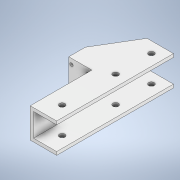
# Autodesk Inventor part: Soporte Linear Rail X
Saved by Autodesk Inventor 2021 (Build 250183000, 183)
## iProperties
Created: 2023-01-21
Part Number: Soporte Linear Rail X
Material: Plástico ABS
Document SubType Name: Modeling
Designer: Diego.labarca
Density: 1.06 g/cm^3
Appearance: Suave - Blanco
Author: Diego.labarca
Autodesk Inventor part; units mm, degrees
ref_plane "YZ Plane" through (0, 0, 0) normal (1, 0, 0) x (0, 1, 0)
ref_plane "XZ Plane" through (0, 0, 0) normal (0, 1, 0) x (-1, 0, 0)
ref_plane "XY Plane" through (0, 0, 0) normal (0, 0, 1) x (1, 0, 0)
sketch "Boceto1" plane through (0, 0, 0) normal (0, 0, 1) x (1, 0, 0)
  line L0 (-10, 11) -> (10, 11)
  line L1 (10, 11) -> (10, -11)
  line L2 (10, -11) -> (-10, -11)
  line L3 (-10, -11) -> (-10, 11)
  line L4 (1.6972, 0) -> (0, 0)
  line L5 (0, 0) -> (0, 1.3941)
  dimension "d11" = 22
  dimension "d12" = 20
  constraints: 12 end point, 2 horizontal, 2 parallel, 2 perpendicular, 2 other
  measures "d11" distance of L0.end L1.end
  measures "d12" distance of L0.start L0.end
extrude "Extrusión1" add sketch "Boceto1" along normal blind 15
sketch "Boceto5" plane through (0, 0, 15) normal (0, 0, 1) x (1, 0, 0)
  line L0 (-10, -11) -> (10, -11) projected
  line L1 (-10, -11) -> (35, -11)
  line L2 (35, -11) -> (35, -14)
  line L3 (35, -14) -> (-10, -14)
  line L4 (-10, -14) -> (-10, -11)
  line L5 (10, -11) -> (10, 11) projected
  line L6 (-10, 11) -> (-10, -11) projected
  line L7 (-10, 10) -> (35, 10)
  line L8 (35, 10) -> (35, 13)
  line L9 (35, 13) -> (-10, 13)
  line L10 (-10, 13) -> (-10, 10)
  line L11 (10, 11) -> (-10, 11) projected
  point P0 (0, 0)
  point P1 (10, 10)
  dimension "d25" = 3
  dimension "d26" = 25
  dimension "d28" = 3
  dimension "d29" = 1
  constraints: 16 end point, 4 parallel, 2 horizontal, 2 perpendicular, 1 collinear, 1 point on line
  measures "d25" distance of L1.end L2.end
  measures "d26" distance between parallel lines of L5 L2
  measures "d28" distance of L8.end L7.end
  measures "d29" distance from line of L7.start L11
extrude "Extrusión5" add sketch "Boceto5" against normal up to surface (15 mm away) contours L0 L1 L2 L3 L4 | L5 L11 L10 L9 L8 L7
sketch "Boceto7" plane through (0, 0, 0) normal (0, 0, -1) x (-1, 0, 0)
  line L0 (10, 13) -> (-35, 13) projected
  line L1 (-35, 10) -> (-10, 10) projected
  line L2 (-35, 13) -> (-15, 13)
  line L3 (-15, 13) -> (-15, 10)
  line L4 (-15, 10) -> (-35, 10)
  line L5 (-35, 10) -> (-35, 13)
  line L6 (-10, -11) -> (-35, -11) projected
  line L7 (-35, -14) -> (10, -14) projected
  line L8 (-35, -11) -> (-15, -11)
  line L9 (-15, -11) -> (-15, -14)
  line L10 (-15, -14) -> (-35, -14)
  line L11 (-35, -14) -> (-35, -11)
  point P0 (0, 0)
  dimension "d32" = 20
  constraints: 16 end point, 4 parallel, 3 point on line, 2 horizontal, 2 perpendicular
  measures "d32" distance of L3.end L4.end
extrude "Extrusión6" add sketch "Boceto7" along normal blind 35 and the other way blind 71
ref_plane "Plano de trabajo1" through (0, 0, 7.5) normal (0, 0, -1) x (-1, 0, 0)
sketch "Boceto10" plane through (0, 0, -35) normal (0, 0, -1) x (-1, 0, 0)
  line L0 (10, 13) -> (-15, 13) projected
  line L1 (-10, 10) -> (-15, 10) projected
  line L2 (-15, 13) -> (-14, 13)
  line L3 (-14, 13) -> (-14, 10)
  line L4 (-14, 10) -> (-15, 10)
  line L5 (-15, 10) -> (-15, 13)
  line L6 (-15, -14) -> (-15, -11) projected
  line L7 (10, -14) -> (-15, -14) projected
  line L8 (-15, -11) -> (-14, -11)
  line L9 (-14, -11) -> (-14, -14)
  line L10 (-14, -14) -> (-15, -14)
  line L11 (-15, -14) -> (-15, -11)
  line L12 (-14, -14) -> (-11, -14)
  line L13 (-11, -14) -> (-11, 13)
  line L14 (-11, 13) -> (-14, 13)
  line L15 (-14, 13) -> (-14, -14)
  point P0 (0, 0)
  point P1 (-11, 10)
  dimension "d60" = 1
  dimension "d61" = 1
  dimension "d62" = 3
  constraints: 24 end point, 6 parallel, 3 horizontal, 3 perpendicular, 3 point on line
  measures "d60" distance of L3.end L4.end
  measures "d61" distance of L9.end L10.end
  measures "d62" distance of L14.end L13.end
extrude "Extrusión9" add sketch "Boceto10" against normal up to surface (106 mm away)
sketch "Boceto11" plane through (-10, 13, 15) normal (0, 1, 0) x (1, 0, 0)
  line L0 (0, 0) -> (0, 15) projected
  circle A0 centre (35, 7.5) radius 2.5
  circle A1 centre (35, 40) radius 2.5
  circle A2 centre (35, -41) radius 2.5
  line L1 (21, 50) -> (45, 50) projected
  line L2 (45, -56) -> (21, -56) projected
  line L3 (45, -56) -> (45, 50) projected
  point P0 (10, 15)
  dimension "d65" = 5
  dimension "d66" = 5
  dimension "d67" = 5
  dimension "d69" = 10
  dimension "d70" = 15
  dimension "d73" = 10
  dimension "d74" = 10
  dimension "d75" = 10
  constraints: 3 centre point
  measures "d65" diameter of A0
  measures "d66" diameter of A2
  measures "d67" diameter of A1
  measures "d69" distance from line of A1.centre L1
  measures "d70" distance from line of L2 A2.centre
  measures "d73" distance from line of L3 A2.centre
  measures "d74" distance from line of L3 A0.centre
  measures "d75" distance from line of L3 A1.centre
extrude "Extrusión10" cut sketch "Boceto11" against normal up to surface (27 mm away)
sketch "Boceto13" plane through (0, 0, 0) normal (0, 0, -1) x (-1, 0, 0)
  line L0 (-10, -11) -> (-10, 10) projected
  line L1 (-11, 10) -> (-10, 10) projected
  line L2 (-10, -11) -> (-11, -11) projected
  line L3 (-11, -14) -> (-11, 13) projected
  point P0 (0, 0)
extrude "Extrusión12" add sketch "Boceto13" against normal up to surface (15 mm away)
sketch "Boceto14" plane through (-10, 13, 15) normal (0, 1, 0) x (1, 0, 0)
  line L0 (21, 50) -> (45, 50) projected
  line L1 (0, 15) -> (21, 50)
  line L2 (21, 50) -> (21, 15) projected
  line L3 (0, 15) -> (21, 15) projected
  point P0 (10, 15)
  constraints: 2 end point
extrude "Extrusión13" add sketch "Boceto14" against normal up to surface (27 mm away)
sketch "Boceto12" plane through (11, -14, -35) normal (-1, 0, 0) x (0, 0, 1)
  circle A0 centre (15, 14) radius 2.5
  line L0 (0, 27) -> (35, 27) projected
  line L1 (0, 0) -> (0, 27) projected
  circle A1 centre (80, 14) radius 2.5
  line L2 (50, 27) -> (106, 27) projected
  line L3 (50, 27) -> (50, 0) projected
  line L4 (106, 0) -> (106, 27) projected
  point P0 (35, 14)
  dimension "d76" = 5
  dimension "d77" = 13
  dimension "d78" = 15
  dimension "d79" = 5
  dimension "d80" = 13
  dimension "d84" = 26
  constraints: 2 centre point
  measures "d76" diameter of A0
  measures "d77" distance from line of L0 A0.centre
  measures "d78" distance from line of L1 A0.centre
  measures "d79" diameter of A1
  measures "d80" distance from line of A1.centre L2
  measures "d84" distance from line of L4 A1.centre
extrude "Extrusión11" cut sketch "Boceto12" against normal through all both and the other way through all
sketch "Boceto15" plane through (-10, -14, 15) normal (-1, 0, 0) x (0, 0, 1)
  circle A0 centre (-35, 14) radius 2.5 projected
  circle A1 centre (-35, 14) radius 2.5 projected
  circle A2 centre (-35, 14) radius 5
  point P0 (-15, 14)
  dimension "d90" = 10
  constraints: 1 centre point, 1 coincident
  measures "d90" diameter of A2
extrude "Extrusión14" cut sketch "Boceto15" against normal blind 14 contours A0 | A2
sketch "Boceto16" plane through (0, 0, 15) normal (0, 0, 1) x (1, 0, 0)
  line L0 (2.28, 0) -> (0, 0)
  line L1 (0, 0) -> (0, 2.8237)
  circle A0 centre (7.5, 8) radius 1.5
  dimension "d93" = 8
  dimension "d94" = 7.5
  dimension "d113" = 3
  constraints: 4 end point, 1 centre point, 1 horizontal, 1 perpendicular
  measures "d93" distance from line of L0 A0.centre
  measures "d94" distance from line of L1 A0.centre
  measures "d113" diameter of A0
extrude "Extrusión15" cut sketch "Boceto16" against normal through all
pattern_linear "Patrón rectangular1" count 2 spacing 15 along (-1, 0, 0) count 2 spacing 16 along (0, -1, 0) of "Extrusión15"
ref_plane "Plano de trabajo2" through (0, 0, -2.5) normal (0, 0, 1) x (1, 0, 0)
sketch "Boceto17" plane through (0, 0, -2.5) normal (0, 0, 1) x (1, 0, 0)
  circle A0 centre (-7.5, 8) radius 1.5 projected
  circle A1 centre (-7.5, -8) radius 1.5 projected
  circle A2 centre (7.5, -8) radius 1.5 projected
  circle A3 centre (7.5, 8) radius 1.5 projected
  circle A4 centre (-7.5, 8) radius 3
  circle A5 centre (-7.5, -8) radius 3
  circle A6 centre (7.5, -8) radius 3
  circle A7 centre (7.5, 8) radius 3
  point P0 (0, 0)
  dimension "d104" = 6
  dimension "d105" = 6
  dimension "d106" = 6
  dimension "d107" = 6
  constraints: 4 centre point, 4 coincident
  measures "d104" diameter of A4
  measures "d105" diameter of A5
  measures "d106" diameter of A6
  measures "d107" diameter of A7
extrude "Extrusión16" cut sketch "Boceto17" against normal up to surface (32.5 mm away) contours A4 | A5
chamfer "Chaflán1" distance 1 angle 45 1 edges at (11, 0, 42.5)
ref_plane "Plano de trabajo3" through (0, 0, -12.5) normal (0, 0, 1) x (1, 0, 0)
sketch "Boceto18" plane through (0, 0, -12.5) normal (0, 0, 1) x (1, 0, 0)
  circle A0 centre (7.5, -8) radius 1.5 projected
  circle A1 centre (7.5, 8) radius 1.5 projected
  circle A2 centre (7.5, -8) radius 3
  circle A3 centre (7.5, 8) radius 3
  dimension "d115" = 6
  dimension "d116" = 6
  constraints: 2 centre point, 2 coincident
  measures "d115" diameter of A2
  measures "d116" diameter of A3
extrude "Extrusión17" cut sketch "Boceto18" against normal up to surface (22.5 mm away)
equation "\"d66\" = d65"
equation "\"d67\" = d65"
equation "\"d74\" = d73"
equation "\"d75\" = d73"
equation "\"d79\" = d76"
equation "\"d80\" = d77"
equation "\"d105\" = d104"
equation "\"d106\" = d104"
equation "\"d107\" = d104"
